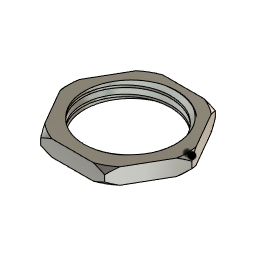
M12x1 nut (Autodesk Fusion 360 design; units mm, degrees)
Autodesk Fusion 360 part; units mm, degrees
sketch "Sketch1" plane through (0, 0, 0) normal (0, 0, 1) x (1, 0, 0)
  circle A0 centre (0, 0) radius 6
  line L0 (8, 0) -> (4, 6.9282)
  line L1 (4, 6.9282) -> (-4, 6.9282)
  line L2 (-4, 6.9282) -> (-8, 0)
  line L3 (-8, 0) -> (-4, -6.9282)
  line L4 (-4, -6.9282) -> (4, -6.9282)
  line L5 (4, -6.9282) -> (8, 0)
  dimension "d1" = 12
  dimension "d2" = 8
  constraint coincident A0.centre origin
  measures "d1" diameter of A0
  measures "d2" distance of L0.start A0.centre
extrude "Extrude1" add sketch "Sketch1" along normal blind 2
thread "Thread1" "ISO Metric profile 12.0 M12x1 6H" major diameter 12.152 minor diameter 11.035 pitch 1 angle 60 modelled right hand crest width 0.2719 on face at (5.9925, -0.2991, 1.3333) crest through (5.5175, 0, 0.25)
sketch "Sketch4" plane through (0, 0, 2) normal (0, 0, 1) x (-1, 0, 0)
  line L0 (-8, 0) -> (-7.4, 0) construction
  point P0 (-8, 0)
  dimension "d5" = 0.6
  constraint coincident P0 L0.start
  constraint horizontal L0
  measures "d5" distance of P0 L0.end
sketch "Sketch5" plane through (0, 0, 0) normal (0, 1, 0) x (1, 0, 0)
  line L0 (4, 0) -> (4, -2) construction
  line L1 (4, -1) -> (9.4, -1) construction
  line L2 (8, 0) -> (8, -2)
  line L3 (7.4, -2) -> (8, -2)
  line L4 (7.4, -2) -> (8, -1.4)
  line L5 (7.4, 0) -> (8, 0)
  line L6 (7.4, 0) -> (8, -0.6)
  line L7 (0, 0) -> (0, -3.5) construction
  point P0 (7.4, -2)
  point P1 (8, 0)
  point P2 (7.4, 0)
  constraint midpoint L0 L1.start
  constraint perpendicular L0 L1
  constraint coincident P0 L3.start
  constraint coincident L2.end L3.end
  constraint coincident L2 L4.end
  constraint symmetric L1 L2.end P1
  constraint symmetric L1 P0 P2
  constraint symmetric L1 L4.end L6.end
  constraint coincident L7.start origin
  constraint vertical L7
revolve "Revolve1" cut sketch "Sketch5" angle 360 about axis through (0, 0, 0) along (0, 0, 1)
